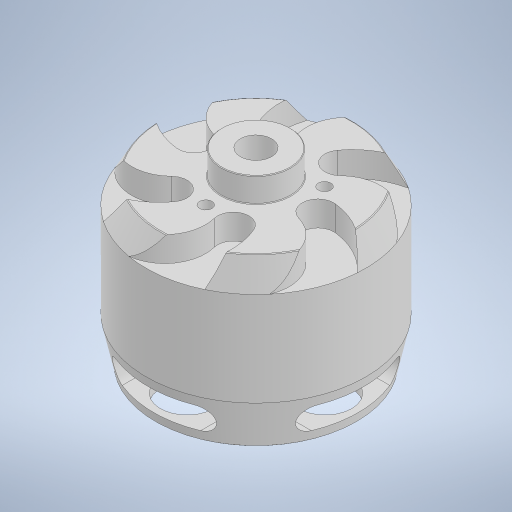
# Autodesk Inventor part: Body - Basic
Saved by Autodesk Inventor 2023.2 (Build 272271000, 271)
## iProperties
Created: 2022-12-15
Part Number: Body - Basic
Material: Generic
Document SubType Name: Modeling
Designer: Nathan Cai
Density: 1 g/cm^3
Appearance: Default
Author: Nathan Cai
Autodesk Inventor part; units mm, degrees
ref_plane "YZ Plane" through (0, 0, 0) normal (1, 0, 0) x (0, 1, 0)
ref_plane "XZ Plane" through (0, 0, 0) normal (0, 1, 0) x (-1, 0, 0)
ref_plane "XY Plane" through (0, 0, 0) normal (0, 0, 1) x (1, 0, 0)
sketch "Sketch1" plane through (0, 0, 0) normal (0, 0, 1) x (1, 0, 0)
  line L0 (0, 0) -> (0, 29.9)
  line L1 (0, 0) -> (16, 0)
  line L2 (0, 7) -> (17.5, 7)
  line L3 (16, 0) -> (17.5, 7)
  line L4 (0, 22) -> (17.5, 22)
  line L5 (17.5, 22) -> (17.5, 7)
  line L6 (0, 26) -> (15.25, 26)
  line L7 (15.25, 26) -> (17.5, 22)
  line L8 (0, 26) -> (5.5, 26)
  line L9 (5.5, 26) -> (5.5, 29.9)
  line L10 (5.5, 29.9) -> (0, 29.9)
  line L11 (0, 29.9) -> (0, 26)
  line L12 (0, 0) -> (2.5, 0)
  line L13 (2.5, 0) -> (2.5, 29.9)
  line L14 (2.5, 29.9) -> (0, 29.9)
  line L15 (0, 29.9) -> (0, 0)
  point P0 (8, 0)
  dimension "d0" = 29.9
  dimension "d1" = 16
  dimension "d2" = 17.5
  dimension "d3" = 7
  dimension "d4" = 22
  dimension "d5" = 15.25
  dimension "d6" = 4
  dimension "d7" = 5.5
  dimension "d8" = 2.5
  constraints: 32 end point, 6 horizontal, 5 point on line, 4 parallel, 3 perpendicular, 1 midpoint, 1 vertical
  measures "d0" distance of L0.start L0.end
  measures "d1" distance of L0.start L1.end
  measures "d2" distance of L2.start L2.end
  measures "d3" distance between parallel lines of L1 L2
  measures "d4" distance from line of point (8, 0) L4
  measures "d5" distance of L6.start L6.end
  measures "d6" distance between parallel lines of L4 L6
  measures "d7" distance of L10.end L9.end
  measures "d8" distance between parallel lines of L0 L13
revolve "Revolution1" add sketch "Sketch1" angle 360 about axis through (0, 29.9, 0) along (0, -1, 0) contours L13 L2 L3 L1 | L13 L4 L5 L2 | L13 L6 L7 L4 | L13 L10 L9 L6
chamfer "Chamfer1" distance 0.1 angle 45 4 edges at (-5.5, 29.9, 0) (-5.5, 26, 0) (-15.25, 26, 0) (-16, 0, 0)
sketch "Sketch2" plane through (0, 26, 0) normal (0, 1, 0) x (1, 0, 0)
  circle A0 centre (0, 0) radius 8 construction
  circle A1 centre (6.9282, 4) radius 1
  circle A2 centre (-6.9282, 4) radius 1
  circle A3 centre (0, -8) radius 1
  line L0 (0, -8) -> (0, 0) construction
  circle A4 centre (0, 0) radius 7.375 construction
  line L1 (0, 0) -> (3.6875, -6.3869) construction
  arc A5 (7.2299, -7.5545) -> (2.5151, -9.1701) centre (4.9375, -8.552) ccw
  arc A6 (7.6002, -15.7635) -> (7.2299, -7.5545) centre (-3.315, -12.1431) ccw
  circle A7 centre (0, 0) radius 17.5
  arc A8 (-3.0379, -17.2343) -> (2.5151, -9.1701) centre (-3.7831, -10.7772) ccw
  circle A9 centre (0, 0) radius 15.25 construction
  circle A10 centre (0, 0) radius 2.5
  circle A11 centre (0, 0) radius 2.5 projected
  line L2 (-3.0379, -17.2343) -> (0, -8) construction
  line L3 (7.6002, -15.7635) -> (4.9375, -8.552) construction
  line L4 (8.1612, -12.8825) -> (-6.9282, 4) construction
  arc A12 (17.4517, -1.2997) -> (10.1573, 2.484) centre (8.8587, -8.9424) ccw
  arc A13 (10.1573, 2.484) -> (9.1991, -2.4069) centre (9.875, 0) ccw
  arc A14 (13.4064, -11.248) -> (9.1991, -2.4069) centre (7.4418, -8.6648) ccw
  arc A15 (9.8514, 14.4637) -> (2.9274, 10.0385) centre (12.1737, 3.2006) ccw
  arc A16 (2.9274, 10.0385) -> (6.684, 6.7632) centre (4.9375, 8.552) ccw
  arc A17 (16.4443, 5.9863) -> (6.684, 6.7632) centre (11.2248, 2.1123) ccw
  arc A18 (-7.6002, 15.7635) -> (-7.2299, 7.5545) centre (3.315, 12.1431) ccw
  arc A19 (-7.2299, 7.5545) -> (-2.5151, 9.1701) centre (-4.9375, 8.552) ccw
  arc A20 (3.0379, 17.2343) -> (-2.5151, 9.1701) centre (3.7831, 10.7772) ccw
  arc A21 (-17.4517, 1.2997) -> (-10.1573, -2.484) centre (-8.8587, 8.9424) ccw
  arc A22 (-10.1573, -2.484) -> (-9.1991, 2.4069) centre (-9.875, 0) ccw
  arc A23 (-13.4064, 11.248) -> (-9.1991, 2.4069) centre (-7.4418, 8.6648) ccw
  arc A24 (-9.8514, -14.4637) -> (-2.9274, -10.0385) centre (-12.1737, -3.2006) ccw
  arc A25 (-2.9274, -10.0385) -> (-6.684, -6.7632) centre (-4.9375, -8.552) ccw
  arc A26 (-16.4443, -5.9863) -> (-6.684, -6.7632) centre (-11.2248, -2.1123) ccw
  point P0 (15.2371, 0.6266)
  point P1 (7.0759, 13.509)
  point P2 (-8.1612, 12.8825)
  point P3 (-15.2371, -0.6266)
  point P4 (-7.0759, -13.509)
  point P5 (13.4064, -11.248)
  point P6 (17.4517, -1.2997)
  point P7 (3.0379, 17.2343)
  point P8 (-7.6002, 15.7635)
  point P9 (-13.4064, 11.248)
  point P10 (-17.4517, 1.2997)
  point P11 (16.4443, 5.9863)
  point P12 (-16.4443, -5.9863)
  dimension "d19" = 14.75
  dimension "d23" = 30.5
  dimension "d13" = 16
  dimension "d14" = 2
  dimension "d17" = 360
  dimension "d21" = 5
  dimension "d22" = 35
  dimension "d24" = 5
  dimension "d26" = 30
  dimension "d27" = 6.5
  dimension "d28" = 11.5
  dimension "d31" = 360
  constraints: 46 point on circle, 24 centre point, 10 end point, 6 coincident, 4 tangent, 1 point on line, 1 vertical, 81 other
  measures "d13" diameter of A0
  measures "d14" diameter of A1
  measures "d21" diameter of A5
  measures "d22" diameter of A7
  measures "d24" diameter of A10
  measures "d26" angle of L0 L1
  measures "d27" radius of A8
  measures "d28" radius of A6
extrude "Extrusion1" cut sketch "Sketch2" against normal blind 4 contours A1 | A2 | A3 | A6 A7 A8 A5 | A14 A13 A12 A7 | A7 A26 A25 A24 | A7 A23 A22 A21 | A17 A16 A15 A7 | A7 A20 A19 A18 | A10
sketch "Sketch3" plane through (0, 0, 0) normal (0, -1, 0) x (1, 0, 0)
  circle A0 centre (0, 0) radius 11 construction
  circle A1 centre (0, 0) radius 9.5 construction
  circle A2 centre (0, 0) radius 12.5 construction
  line L0 (0, 0) -> (11, 0) construction
  circle A3 centre (11, 0) radius 4.25
  circle A4 centre (0, 11) radius 4.25
  circle A5 centre (-11, 0) radius 4.25
  circle A6 centre (0, -11) radius 4.25
  line L1 (0, 0) -> (7.7782, -7.7782) construction
  line L2 (0, 0) -> (11, 0) construction
  circle A7 centre (7.7782, -7.7782) radius 1.5
  line L3 (0, 0) -> (8.8388, 8.8388) construction
  circle A8 centre (8.8388, 8.8388) radius 1.5
  circle A9 centre (-8.8388, -8.8388) radius 1.5
  circle A10 centre (-7.7782, 7.7782) radius 1.5
  dimension "d37" = 25
  dimension "d35" = 22
  dimension "d36" = 19
  dimension "d38" = 8.5
  dimension "d41" = 360
  dimension "d43" = 45
  dimension "d44" = 3
  dimension "d45" = 3
  dimension "d48" = 360
  constraints: 10 centre point, 8 end point, 6 coincident, 2 horizontal, 2 point on circle, 1 equal length, 1 perpendicular, 21 other
  measures "d35" diameter of A0
  measures "d36" diameter of A1
  measures "d38" diameter of A3
  measures "d43" angle of L1 L2
  measures "d44" diameter of A7
  measures "d45" diameter of A8
extrude "Extrusion2" cut sketch "Sketch3" against normal blind 1.5
sketch "Sketch4" plane through (0, 0, 0) normal (0, 0, 1) x (1, 0, 0)
  line L0 (6.25, 3.5) -> (-6.25, 3.5) construction
  line L1 (6.25, 5.5) -> (-6.25, 5.5)
  line L2 (-6.25, 1.5) -> (6.25, 1.5)
  arc A0 (6.25, 1.5) -> (6.25, 5.5) centre (6.25, 3.5) ccw
  arc A1 (-6.25, 5.5) -> (-6.25, 1.5) centre (-6.25, 3.5) ccw
  line L3 (0, 0) -> (0, 29.8) construction
  line L4 (5.5, 29.8) -> (-5.5, 29.8) projected
  line L5 (-2.5, 0) -> (2.5, 0) projected
  point P0 (0, 3.5)
  dimension "d52" = 12.5
  dimension "d53" = 2
  dimension "d54" = 1.5
  constraints: 10 end point, 4 point on circle, 4 tangent, 2 centre point, 2 midpoint, 1 horizontal, 1 parallel, 1 point on line
  measures "d52" distance of L0.start L0.end
  measures "d53" radius of A1
  measures "d54" distance between parallel lines of L5 L2
extrude "Extrusion3" cut sketch "Sketch4" along normal through all both and the other way through all
pattern_circular "Circular Pattern1" count 2 over 90 about axis through (0, 14.5, 0) along (0, -1, 0) of "Extrusion3"
body "Solid1"
